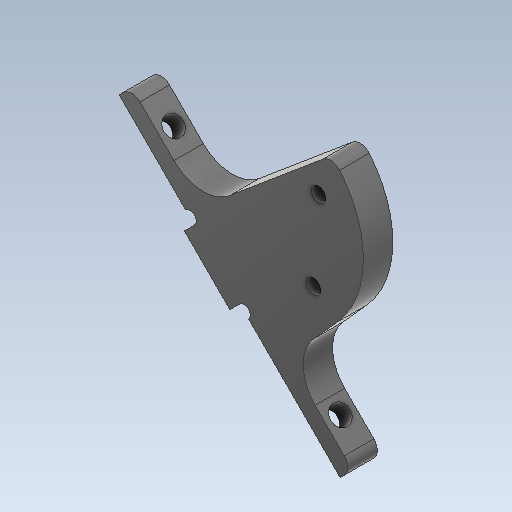
# Autodesk Inventor part: Camera_vertical_frame_01
Saved by Autodesk Inventor 2020.4 (Build 244396000, 396)
## iProperties
Created: 2021-09-02
Part Number: Camera_vertical_frame_01
Material: アセタール樹脂、黒
Document SubType Name: Modeling
Designer: t-nagamine
Density: 1.425 g/cm^3
Appearance: 滑らか - 黒
Author: t-nagamine
Autodesk Inventor part; units mm, degrees
ref_plane "YZ Plane" through (0, 0, 0) normal (1, 0, 0) x (0, 1, 0)
ref_plane "XZ Plane" through (0, 0, 0) normal (0, 1, 0) x (-1, 0, 0)
ref_plane "XY Plane" through (0, 0, 0) normal (0, 0, 1) x (1, 0, 0)
derived "Head_vertical_frame_01.ipt"
sketch "スケッチ1" plane through (0, 0, 0) normal (0, 0, 1) x (1, 0, 0)
  line L0 (0, 0) -> (27, 0) construction
  line L1 (27, 0) -> (27, 5) construction
  line L2 (27, 5) -> (0, 5) construction
  line L3 (0, 5) -> (0, 0) construction
  line L4 (0, 2.5) -> (27, 2.5) construction
  line L5 (13.5, 5) -> (13.5, 0) construction
  circle A0 centre (3.7, 2.5) radius 1.55 projected
  line L6 (7.5, 5) -> (7.5, 0) construction
  line L7 (19.5, 5) -> (19.5, 0) construction
  circle A1 centre (23.3, 2.5) radius 1.55 projected
  line L8 (7.49, 5.01) -> (9.59, 5.01) construction
  line L9 (19.51, 5.01) -> (19.51, -0.01) projected
  line L10 (19.51, -0.01) -> (17.41, -0.01) construction
  line L11 (7.49, -0.01) -> (7.49, 5.01) projected
  line L12 (7.49, 5.01) -> (19.51, -0.01) construction
  line L13 (19.51, 5.01) -> (7.49, -0.01) construction
  line L14 (0, 0) -> (7.5, -3) projected
  line L15 (7.5, -3) -> (19.5, -3) projected
  line L16 (27, 0) -> (19.5, -3) projected
  arc A2 (9.59, 5.01) -> (7.49, 5.01) centre (8.54, 5.01) ccw projected
  arc A3 (7.49, -0.01) -> (9.59, -0.01) centre (8.54, -0.01) ccw projected
  arc A4 (19.51, 5.01) -> (17.41, 5.01) centre (18.46, 5.01) ccw projected
  arc A5 (17.41, -0.01) -> (19.51, -0.01) centre (18.46, -0.01) ccw projected
  line L17 (9.59, 5.01) -> (17.41, 5.01) projected
  line L18 (9.59, -0.01) -> (7.49, -0.01) construction
  line L19 (17.41, 5.01) -> (19.51, 5.01) construction
  line L20 (17.41, -0.01) -> (9.59, -0.01) projected
  line L21 (27, 7) -> (0, 7) construction
  line L22 (0, 0) -> (0, 7) projected
  line L23 (12.1912, 40) -> (12.1912, 35) construction
  circle A6 centre (14.8912, 37.5) radius 1.55 projected
  line L24 (37.1912, 35) -> (37.1912, 40) construction
  line L25 (30.6912, 40) -> (30.6912, 35) construction
  circle A7 centre (34.4912, 37.5) radius 1.55 projected
  line L26 (30.7012, 40.01) -> (30.7012, 34.99) projected
  line L27 (18.6912, 40) -> (18.6912, 35) construction
  line L28 (12.1912, 35) -> (37.1912, 35) construction
  line L29 (37.1912, 40) -> (12.1912, 40) construction
  line L30 (12.1912, 37.5) -> (37.1912, 37.5) construction
  line L31 (24.6912, 40) -> (24.6912, 35) construction
  line L32 (20.7812, 40.01) -> (28.6012, 40.01) projected
  line L33 (28.6012, 34.99) -> (20.7812, 34.99) projected
  line L34 (18.6812, 40.01) -> (30.7012, 34.99) construction
  line L35 (30.7012, 40.01) -> (18.6812, 34.99) construction
  arc A8 (30.7012, 40.01) -> (28.6012, 40.01) centre (29.6512, 40.01) ccw projected
  line L36 (28.6012, 40.01) -> (30.7012, 40.01) construction
  arc A9 (28.6012, 34.99) -> (30.7012, 34.99) centre (29.6512, 34.99) ccw projected
  line L37 (30.7012, 34.99) -> (28.6012, 34.99) construction
  line L38 (18.6812, 40.01) -> (20.7812, 40.01) construction
  line L39 (20.7812, 34.99) -> (18.6812, 34.99) construction
  arc A10 (20.7812, 40.01) -> (18.6812, 40.01) centre (19.7312, 40.01) ccw projected
  arc A11 (18.6812, 34.99) -> (20.7812, 34.99) centre (19.7312, 34.99) ccw projected
  line L40 (18.6812, 34.99) -> (18.6812, 40.01) projected
  line L41 (18.6912, 73) -> (18.6912, 68) construction
  line L42 (18.6812, 67.99) -> (18.6812, 73.01) projected
  line L43 (20.7812, 67.99) -> (18.6812, 67.99) construction
  arc A12 (18.6812, 67.99) -> (20.7812, 67.99) centre (19.7312, 67.99) ccw projected
  arc A13 (20.7812, 73.01) -> (18.6812, 73.01) centre (19.7312, 73.01) ccw projected
  line L44 (24.6912, 73) -> (24.6912, 68) construction
  line L45 (12.1912, 70.5) -> (37.1912, 70.5) construction
  line L46 (37.1912, 73) -> (12.1912, 73) construction
  line L47 (12.1912, 68) -> (37.1912, 68) construction
  line L48 (30.7012, 73.01) -> (18.6812, 67.99) construction
  line L49 (18.6812, 73.01) -> (30.7012, 67.99) construction
  line L50 (28.6012, 67.99) -> (20.7812, 67.99) projected
  line L51 (20.7812, 73.01) -> (28.6012, 73.01) projected
  line L52 (37.1912, 68) -> (37.1912, 73) construction
  line L53 (18.6812, 73.01) -> (20.7812, 73.01) construction
  line L54 (30.6912, 73) -> (30.6912, 68) construction
  arc A14 (30.7012, 73.01) -> (28.6012, 73.01) centre (29.6512, 73.01) ccw projected
  line L55 (28.6012, 73.01) -> (30.7012, 73.01) construction
  line L56 (30.7012, 73.01) -> (30.7012, 67.99) projected
  line L57 (30.7012, 67.99) -> (28.6012, 67.99) construction
  circle A15 centre (34.4912, 70.5) radius 1.55 projected
  arc A16 (28.6012, 67.99) -> (30.7012, 67.99) centre (29.6512, 67.99) ccw projected
  circle A17 centre (14.8912, 70.5) radius 1.55 projected
  line L58 (12.1912, 73) -> (12.1912, 68) construction
  line L59 (27, 0) -> (27, 6.6473) projected
  line L60 (37.1912, 35) -> (27.1206, 7.3314) projected
  line L61 (11.8992, 39.6929) -> (0, 7) projected
  line L62 (37.1912, 35) -> (37.1912, 73) projected
  line L63 (9.1035, 103.3621) -> (4.9463, 99.8738) construction
  arc A18 (3.8121, 84.8933) -> (4.5202, 97.3071) centre (-4.8938, 91.617) ccw construction
  circle A19 centre (-4.8938, 91.617) radius 14.6063 construction
  line L64 (1.0459, 61.9185) -> (-21.5815, 84.5459) construction
  line L65 (-21.5815, 84.5459) -> (-18.0459, 88.0815) construction
  line L66 (-18.0459, 88.0815) -> (4.5815, 65.4541) construction
  line L67 (4.5815, 65.4541) -> (1.0459, 61.9185) construction
  line L68 (1.0459, 61.9185) -> (-18.0459, 88.0815) construction
  line L69 (-21.5815, 84.5459) -> (4.5815, 65.4541) construction
  line L70 (11.9212, 103.1156) -> (37.1912, 73) construction
  arc A20 (11.8992, 39.6929) -> (3.8916, 82.3518) centre (-28.1256, 54.2607) ccw construction
  arc A21 (8.344, 97.7899) -> (6.2953, 101.0057) centre (-4.8938, 91.617) ccw construction
  arc A22 (5.0756, 80.942) -> (7.4988, 83.886) centre (-4.8938, 91.617) ccw construction
  circle A23 centre (8.344, 97.7899) radius 1.65 projected
  circle A24 centre (7.4988, 83.886) radius 1.65 projected
  arc A25 (11.9212, 103.1156) -> (9.1035, 103.3621) centre (10.3891, 101.83) ccw projected
  arc A26 (4.9463, 99.8738) -> (4.5202, 97.3071) centre (6.2318, 98.3417) ccw construction
  arc A27 (3.8121, 84.8933) -> (3.8916, 82.3518) centre (5.395, 83.6708) ccw construction
  arc A28 (11.9212, 103.1156) -> (9.1035, 103.3621) centre (10.3891, 101.83) ccw
  line L71 (-4.9998, 75.0354) -> (-3.5149, 73.5504) construction
  line L72 (-4.9998, 75.0354) -> (-6.6969, 73.3383)
  line L73 (-6.6969, 73.3383) -> (-14.4043, 81.0458)
  line L74 (-14.4043, 81.0458) -> (-12.7073, 82.7428)
  line L75 (-12.7073, 82.7428) -> (-13.4497, 83.4853) construction
  arc A29 (7.5, 76.1359) -> (7.7635, 66.5147) centre (12.7132, 71.4645) ccw
  line L76 (7.5, 76.1359) -> (11.5561, 80.6624)
  line L77 (30.6912, 102.0166) -> (30.7012, 102.0277)
  arc A30 (11.5561, 80.6624) -> (11.9212, 103.1156) centre (-1.2073, 92.0995) ccw
  arc A31 (27.1206, 7.3314) -> (27, 6.6473) centre (29, 6.6473) ccw projected
  line L78 (-25.4706, 95.5061) -> (-24.7635, 96.2132)
  line L79 (-21.935, 96.2132) -> (-16.1963, 90.4745)
  arc A32 (-16.1963, 90.4745) -> (-6.747, 90.0619) centre (-11.2466, 95.4242) ccw
  line L80 (9.1035, 103.3621) -> (-6.747, 90.0619)
  line L81 (12.0061, 58.0294) -> (12.7132, 58.7365)
  line L82 (12.7132, 61.565) -> (7.7635, 66.5147)
  line L83 (-3.5149, 73.5504) -> (12.0061, 58.0294)
  circle A33 centre (8.344, 97.7899) radius 1.25
  circle A34 centre (7.4988, 83.886) radius 1.25
  arc A35 (-3.5149, 73.5504) -> (-4.9998, 75.0354) centre (-4.2574, 74.2929) ccw
  line L84 (12.0061, 58.0294) -> (-25.4706, 95.5061) construction
  line L85 (-25.4706, 95.5061) -> (-14.1922, 84.2277)
  arc A36 (-12.7073, 82.7428) -> (-14.1922, 84.2277) centre (-13.4497, 83.4853) ccw
  arc A37 (-21.935, 96.2132) -> (-24.7635, 96.2132) centre (-23.3492, 94.799) ccw
  arc A38 (12.7132, 58.7365) -> (12.7132, 61.565) centre (11.299, 60.1508) ccw
  point P0 (13.5, 2.5)
  point P1 (24.6912, 37.5)
  point P2 (24.6912, 70.5)
  point P3 (10.6356, 104.6477)
  point P4 (3.5327, 98.6877)
  point P5 (-8.5, 75)
  point P6 (14.1274, 60.1508)
  dimension "d15" = 2.4
  dimension "d16" = 10.9
  dimension "d17" = 2.4
  dimension "d49" = 7
  dimension "d67" = 7
  dimension "d71" = 3
  dimension "d72" = 9
  dimension "d73" = 53
  dimension "d75" = 17.138
  dimension "d76" = 2.5
  dimension "d77" = 2.5
  dimension "d81" = 15.95
  dimension "d82" = 1.05
  dimension "d83" = 3
  dimension "d84" = 10.5
  dimension "d85" = 1.05
  dimension "d86" = 2
  constraints: 30 end point, 16 point on circle, 15 tangent, 10 centre point, 7 perpendicular, 7 point on line, 2 coincident, 2 equal radius, 1 collinear, 1 line through centre, 1 parallel
  measures "d15" distance of L71.start L72.end
  measures "d16" distance of L72.end L73.end
  measures "d17" distance of L73.end L74.end
  measures "d49" radius of A29
  measures "d67" radius of A32
  measures "d71" distance of L81.start point (14.127, 60.151)
  measures "d72" distance of point (14.127, 60.151) L82.end
  measures "d73" distance between parallel lines of L78 L81
  measures "d75" radius of A30
  measures "d76" diameter of A33
  measures "d77" diameter of A34
  measures "d81" distance of L78.start L85.end
  measures "d82" radius of A36
  measures "d83" distance between parallel lines of L85 L79
  measures "d84" distance between parallel lines of L81 L67
  measures "d85" radius of A35
  measures "d86" radius of A37
extrude "押し出し6" add sketch "スケッチ1" against normal blind 5 contours A23 | A24 | A30 L76 A29 L82 A38 L81 L83 A35 L72 L73 L74 A36 L85 L78 A37 L79 A32 L80 A25
sketch "スケッチ5" plane through (-25.4706, 95.5061, 0) normal (-0.7071068, -0.7071068, 0) x (-0.7071068, 0.7071068, 0)
  circle A0 centre (-6.5, 2.5) radius 1.65
  circle A1 centre (-46.5, 2.5) radius 1.65
  line L0 (0, 0) -> (0, 5) projected
  line L1 (0, 0) -> (-15.95, 0) projected
  line L2 (-53, 0) -> (-53, 5) projected
  line L3 (-31.05, 0) -> (-53, 0) projected
  point P0 (-85.5434, 0)
  dimension "d89" = 3.3
  dimension "d90" = 3.3
  dimension "d91" = 6.5
  dimension "d92" = 2.5
  dimension "d93" = 6.5
  dimension "d94" = 2.5
  constraints: 2 centre point
  measures "d89" diameter of A0
  measures "d90" diameter of A1
  measures "d91" distance from line of L0 A0.centre
  measures "d92" distance from line of L1 A0.centre
  measures "d93" distance from line of L2 A1.centre
  measures "d94" distance from line of L3 A1.centre
extrude "押し出し7" cut sketch "スケッチ5" against normal through all
